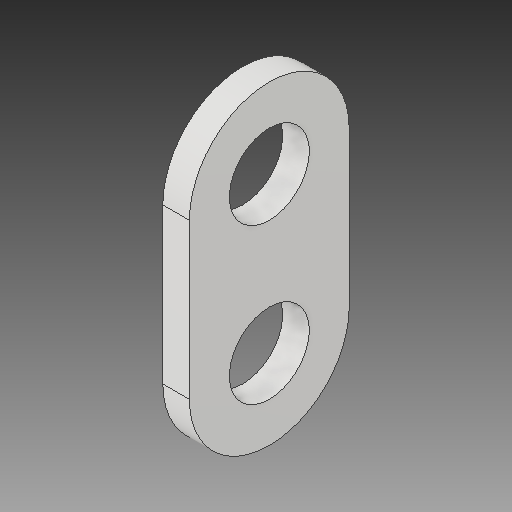
# Autodesk Inventor part: Dummy_JointPosiion
Saved by Autodesk Inventor 2018.3 (Build 223284000, 284)
## iProperties
Created: 2018-02-15
Part Number: Dummy_JointPosiion
Material: ABS プラスチック
Document SubType Name: Modeling
Designer: sktom
Density: 1.06 g/cm^3
Appearance: 滑らか - 白
Author: sktom
Autodesk Inventor part; units mm, degrees
ref_plane "YZ Plane" through (0, 0, 0) normal (1, 0, 0) x (0, 1, 0)
ref_plane "XZ Plane" through (0, 0, 0) normal (0, 1, 0) x (-1, 0, 0)
ref_plane "XY Plane" through (0, 0, 0) normal (0, 0, 1) x (1, 0, 0)
sketch "スケッチ1" plane through (0, 0, 0) normal (1, 0, 0) x (0, 1, 0)
  circle A0 centre (0, 0) radius 1.5
  circle A1 centre (5.823, 0) radius 1.5
  line L0 (0, 0) -> (5.823, 0) construction
  line L1 (0, -3) -> (5.823, -3)
  line L2 (5.823, 3) -> (0, 3)
  arc A2 (0, 3) -> (0, -3) centre (0, 0) ccw
  arc A3 (5.823, -3) -> (5.823, 3) centre (5.823, 0) ccw
  point P0 (2.9115, 0)
  dimension "d0" = 3
  dimension "d1" = 5.823
  dimension "d2" = 3
  constraints: 8 end point, 4 centre point, 4 point on circle, 4 tangent, 1 coincident, 1 equal radius, 1 horizontal, 1 horizontal alignment, 1 midpoint, 1 parallel
  measures "d0" diameter of A0
  measures "d1" distance of point (0, 0) L0.end
  measures "d2" radius of A3
extrude "押し出し1" add sketch "スケッチ1" along normal mid plane 1
